J5 (Autodesk Fusion 360 design; units mm, degrees)
part number: 2026-05-30-23-32-57-845
Autodesk Fusion 360 part; units mm, degrees
sketch "Sketch1" plane through (0, 0, 0) normal (0, 0, 1) x (1, 0, 0)
  circle A0 centre (0, 0) radius 3.75
  dimension "d1" = 7.5
  constraint coincident A0.centre origin
  measures "d1" diameter of A0
extrude "Extrude1" add sketch "Sketch1" along normal blind 11
sketch "Sketch2" plane through (0, 0, 11) normal (0, 0, 1) x (-1, 0, 0)
  circle A0 centre (0, 0) radius 3.75
  circle A1 centre (0, 0) radius 4.5
  dimension "d4" = 9
  constraint coincident A0.centre A1.centre
  measures "d4" diameter of A1
extrude "Extrude2" add sketch "Sketch2" along normal blind 2 contours A0 | A1
sketch "Sketch3" plane through (0, 0, 13) normal (0, 0, 1) x (-1, 0, 0)
  circle A0 centre (0, 0) radius 4.5
  line L0 (-1, 3) -> (1, 3)
  line L1 (1, -3) -> (-1, -3)
  line L2 (-3, 1) -> (-3, -1)
  line L3 (3, -1) -> (3, 1)
  line L4 (3, 1) -> (1, 1)
  line L5 (-1, 1) -> (-3, 1)
  line L6 (-1, -3) -> (-1, -1)
  line L7 (-1, 1) -> (-1, 3)
  line L8 (1, 3) -> (1, 1)
  line L9 (1, -1) -> (1, -3)
  line L10 (-3, -1) -> (-1, -1)
  line L11 (1, -1) -> (3, -1)
  dimension "d7" = 6
  dimension "d8" = 6
  dimension "d9" = 2
  constraint horizontal L0
  constraint vertical L8
  constraint horizontal L1
  constraint vertical L6
  constraint horizontal L4
  constraint vertical L2
  constraint horizontal L10
  constraint vertical L3
  constraint collinear L4 L5
  constraint collinear L6 L7
  constraint collinear L8 L9
  constraint collinear L10 L11
  measures "d7" distance of L0.start L1.end
  measures "d8" distance of L3.end L2.start
  measures "d9" distance of L3.end L3.start
extrude "Extrude3" add sketch "Sketch3" along normal blind 21 contours L0 L1 L2 L3 L4 L5 L6 L7 L8 L9 L10 L11
